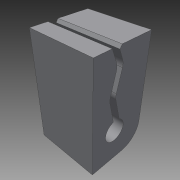
# Autodesk Inventor part: BagClip
Saved by Autodesk Inventor 2015 (Build 190159000, 159)
## iProperties
Created: 2020-03-25
Part Number: BagClip
Material: Generic
Document SubType Name: Modeling
Designer: Dominick Lee
Density: 1 g/cm^3
Appearance: Default
Author: Dominick Lee
Autodesk Inventor part; units mm, degrees
ref_plane "YZ Plane" through (0, 0, 0) normal (1, 0, 0) x (0, 1, 0)
ref_plane "XZ Plane" through (0, 0, 0) normal (0, 1, 0) x (-1, 0, 0)
ref_plane "XY Plane" through (0, 0, 0) normal (0, 0, 1) x (1, 0, 0)
sketch "Sketch1" plane through (0, 0, 0) normal (0, 1, 0) x (-1, 0, 0)
  line L0 (3, 5) -> (-3, 5)
  line L1 (-3, 5) -> (-3, -5)
  line L2 (-3, -5) -> (3, -5)
  line L3 (3, -5) -> (3, 5)
  line L4 (3, 5) -> (-3, -5) construction
  line L5 (-3, 5) -> (3, -5) construction
  point P0 (0, 0)
  dimension "d0" = 6
  dimension "d1" = 10
  constraints: 12 end point, 2 midpoint, 2 parallel, 1 horizontal, 1 perpendicular
  measures "d0" distance of L0.start L0.end
  measures "d1" distance of L1.end L0.end
extrude "Extrusion1" add sketch "Sketch1" along normal blind 5.5
sketch "Sketch2" plane through (-3, 0, -5) normal (-1, 0, 0) x (0, 0, 1)
  line L0 (0, 0) -> (0, 5.5) projected
  line L1 (0, 5.5) -> (10, 5.5) projected
  line L2 (5, 0) -> (6.2, 0)
  line L3 (0, 0) -> (10, 0) projected
  line L4 (6.2, 0) -> (7.4, 0)
  line L5 (7.4, 0) -> (8.6, 0)
  line L6 (6.2, 2.1605) -> (8.6, 2.75)
  line L7 (8.6, 2.75) -> (9.7251, 2.2762)
  line L8 (6.2, 2.1605) -> (6.2, 1.5605)
  line L9 (6.2, 1.5605) -> (3.9766, 2.1182)
  line L10 (6.2, 1.5605) -> (8.6, 2.1605)
  line L11 (8.6, 2.1605) -> (10, 1.5605)
  line L12 (0, 2.3333) -> (3, 2.3333)
  arc A0 (3.8957, 2.7779) -> (3.9766, 2.1182) centre (3, 2.3333) ccw
  line L13 (6.2, 2.1605) -> (3.8957, 2.7779)
  line L14 (6.2, 2.1605) -> (8.5856, 2.1605) construction
  line L15 (9.7251, 2.2762) -> (10, 2.4692)
  line L16 (10, 2.4692) -> (10, 1.5605)
  point P0 (10, 2.3333)
  dimension "d8" = 1.2
  dimension "d9" = 1.2
  dimension "d10" = 1.2
  dimension "d17" = 0.6
  dimension "d18" = 3
  dimension "d19" = 2
  dimension "d20" = 165
  constraints: 28 end point, 4 point on line, 2 horizontal, 2 point on circle, 2 vertical, 1 centre point, 1 coincident, 1 equal length
  measures "d8" distance of L2.start L2.end
  measures "d9" distance of L2.end L4.end
  measures "d10" distance of L4.end L5.end
  measures "d17" distance of L6.start L8.end
  measures "d18" distance of L12.start L12.end
  measures "d19" diameter of A0
  measures "d20" angle of L14 L13
extrude "Extrusion2" cut sketch "Sketch2" against normal blind 6.5
fillet "Fillet2" radius 2 1 edges at (0, 5.5, -5)
fillet "Fillet3" radius 1 4 edges at (0, 2.1605, 3.6) (0, 2.1605, 1.2) (0, 1.5605, 1.2) (0, 2.75, 3.6)
body "Solid1"
